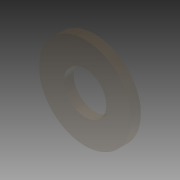
# Autodesk Inventor part: Plastic Washer
Saved by Autodesk Inventor 2013 (Build 170138000, 138)
## iProperties
Created: 2005-07-31
Part Number: Plastic Washer
Document SubType Name: Modeling
Designer: Luke
Density: 1 g/cm^3
Material: Generic
Author: Luke
Autodesk Inventor part; units mm, degrees
ref_plane "YZ Plane" through (0, 0, 0) normal (1, 0, 0) x (0, 1, 0)
ref_plane "XZ Plane" through (0, 0, 0) normal (0, 1, 0) x (-1, 0, 0)
ref_plane "XY Plane" through (0, 0, 0) normal (0, 0, 1) x (1, 0, 0)
sketch "Sketch1" plane through (0, 0, 0) normal (0, 0, 1) x (1, 0, 0)
  circle A0 centre (-13.6107, 11.1425) radius 4.7625
  circle A1 centre (-13.6107, 11.1425) radius 2.1971
  dimension "d0" = 9.525
  dimension "d1" = 4.3942
  constraints: 2 centre point, 1 coincident
  measures "d0" diameter of A0
  measures "d1" diameter of A1
extrude "Extrusion1" add sketch "Sketch1" along normal blind 1.016
body "Solid1"
